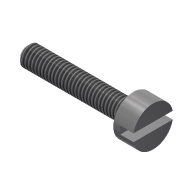
# Autodesk Inventor part: screw_M3-10
Saved by Autodesk Inventor 2015 SP1 (Build 190203100, 203)
## iProperties
Created: 2015-10-09
Part Number: screw_M3-10
Material: Сталь, легированная
Document SubType Name: Modeling
Designer: User
Density: 7.73 g/cm^3
Appearance: С умеренной полировкой
Mass: 1.41584 g
Surface Area: 2.79736 cm^2
Volume: 0.183161 cm^3
Author: User
Autodesk Inventor part; units mm, degrees
ref_plane "YZ Plane" through (0, 0, 0) normal (1, 0, 0) x (0, 1, 0)
ref_plane "XZ Plane" through (0, 0, 0) normal (0, 1, 0) x (-1, 0, 0)
ref_plane "XY Plane" through (0, 0, 0) normal (0, 0, 1) x (1, 0, 0)
sketch "Sketch1" plane through (0, 0, 0) normal (1, 0, 0) x (0, 1, 0)
  circle A0 centre (0, 0) radius 1.5
  circle A1 centre (0, 0) radius 3
  dimension "d0" = 3
  dimension "d1" = 6
  constraints: 2 centre point, 2 coincident
  measures "d0" diameter of A0
  measures "d1" diameter of A1
extrude "Extrusion1" add sketch "Sketch1" against normal blind 16 contours A0
extrude "Extrusion2" add sketch "Sketch1" along normal blind 3 contours A0 | A1
sketch "Sketch2" plane through (3, 0, 0) normal (1, 0, 0) x (0, 0, -1)
  circle A0 centre (0, 0) radius 3 projected
  circle A1 centre (0, 0) radius 3 projected
  line L0 (-0.5749, -2.9444) -> (-0.5749, 2.9444)
  line L1 (0.5749, -2.9444) -> (0.5749, 2.9444)
  line L2 (0, 0) -> (0, 3)
  constraints: 7 point on circle, 6 end point, 3 vertical, 1 other
extrude "Extrusion3" cut sketch "Sketch2" against normal blind 2 contours L1 A0 L0
chamfer "Chamfer1" distance 0.5 angle 45 1 edges at (-16, -1.5, 0)
thread "Thread2" size "M3x0.5" class "6g" standard "ANSI Metric M Profile" full length
body "Solid1"
